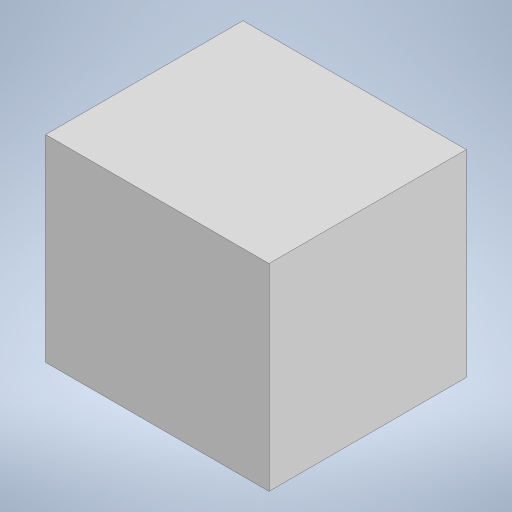
# Autodesk Inventor part: MotorBlock
Saved by Autodesk Inventor 2023 (Build 270158000, 158)
## iProperties
Created: 2024-02-23
Part Number: MotorBlock
Material: Generisch
Document SubType Name: Modeling
Designer: phili
Density: 1 g/cm^3
Appearance: Vorgabe
Author: phili
Autodesk Inventor part; units mm, degrees
ref_plane "YZ Plane" through (0, 0, 0) normal (1, 0, 0) x (0, 1, 0)
ref_plane "XZ Plane" through (0, 0, 0) normal (0, 1, 0) x (-1, 0, 0)
ref_plane "XY Plane" through (0, 0, 0) normal (0, 0, 1) x (1, 0, 0)
sketch "Skizze1" plane through (0, 0, 0) normal (1, 0, 0) x (0, 1, 0)
  line L0 (-13.25, -13.25) -> (13.25, -13.25)
  line L1 (13.25, -13.25) -> (13.25, 13.25)
  line L2 (13.25, 13.25) -> (-13.25, 13.25)
  line L3 (-13.25, 13.25) -> (-13.25, -13.25)
  line L4 (-13.25, -13.25) -> (13.25, 13.25) construction
  line L5 (13.25, -13.25) -> (-13.25, 13.25) construction
  point P0 (0, 0)
  dimension "d0" = 26.5
  dimension "d1" = 26.5
  constraints: 12 end point, 2 midpoint, 2 parallel, 1 horizontal, 1 perpendicular
  measures "d0" distance of L2.end L1.end
  measures "d1" distance of L1.end L0.end
extrude "Extrusion1" add sketch "Skizze1" along normal blind 30
